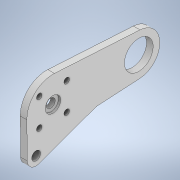
# Autodesk Inventor part: right_wall
Saved by Autodesk Inventor 2020 (Build 240168000, 168)
## iProperties
Created: 2024-02-19
Part Number: right_wall
Material: Типовые
Document SubType Name: Modeling
Designer: 4s
Density: 1 g/cm^3
Appearance: По умолчанию
Author: 4s
Autodesk Inventor part; units mm, degrees
ref_plane "YZ Plane" through (0, 0, 0) normal (1, 0, 0) x (0, 1, 0)
ref_plane "XZ Plane" through (0, 0, 0) normal (0, 1, 0) x (-1, 0, 0)
ref_plane "XY Plane" through (0, 0, 0) normal (0, 0, 1) x (1, 0, 0)
sketch "Эскиз1" plane through (0, 0, 0) normal (1, 0, 0) x (0, 1, 0)
  circle A0 centre (35.2311, -22.6062) radius 9.3
  circle A1 centre (0, -38.8201) radius 6.1
  circle A2 centre (0, 0) radius 4.85
  circle A3 centre (35.8147, -49.5529) radius 3.55
  line L0 (6.0968, -38.6237) -> (4.8475, 0.1562)
  line L1 (-4.8475, 0.1562) -> (-6.0968, -38.6237)
  line L2 (0, 0) -> (0, -38.8201) construction
  circle A4 centre (0, -38.8201) radius 6.5
  circle A5 centre (0, 0) radius 2
  circle A6 centre (0, -38.8201) radius 15 construction
  circle A7 centre (0, 0) radius 14 construction
  circle A8 centre (0, -38.8201) radius 9.5
  circle A9 centre (0, 0) radius 7
  line L3 (9.4833, -39.383) -> (11.7793, -0.6991)
  line L4 (-9.4833, -39.383) -> (-11.7793, -0.6991)
  circle A10 centre (0, 0) radius 8.8
  circle A11 centre (0, 0) radius 11.8
  point P0 (-7, 0)
  point P1 (-9.4833, -39.383)
  point P2 (-11.7793, -0.6991)
  dimension "d27" = 19
  dimension "d0" = 18.6
  dimension "d1" = 12.2
  dimension "d2" = 9.7
  dimension "d3" = 7.1
  dimension "d8" = 38.8201
  dimension "d13" = 38.8
  dimension "d14" = 38.8
  dimension "d23" = 13
  dimension "d24" = 4
  dimension "d25" = 30
  dimension "d26" = 28
  dimension "d28" = 14
  dimension "d31" = 17.6
  dimension "d32" = 3
  constraints: 10 centre point, 10 end point, 9 coincident, 4 point on circle, 4 tangent, 2 symmetric about line, 1 vertical, 8 other
  measures "d0" diameter of A0
  measures "d1" diameter of A1
  measures "d2" diameter of A2
  measures "d3" diameter of A3
  measures "d8" distance of L2.end L2.start
  measures "d13" distance of L0.start L0.end
  measures "d14" distance of L1.start L1.end
  measures "d23" diameter of A4
  measures "d24" diameter of A5
  measures "d25" diameter of A6
  measures "d26" diameter of A7
  measures "d28" diameter of A9
  measures "d31" diameter of A10
extrude "Выдавливание4" add sketch "Эскиз1" along normal blind 3 contours A4 L1 A8 L0 | L0 A8 L1 A4 | A8 L1 A11 L0 | L0 A11 L3 A8 | A8 L4 A11 L1 | A11 L1 A10 L0 | L0 A10 L1 A11 | A10 L1 A9 L0 | L0 A9 L1 A10 | A9 L1 A2 L0 | L0 A2 L1 A9 | A2
sketch "Эскиз4" plane through (0, 0, 0) normal (-1, 0, 0) x (0, 0, 1)
  circle A0 centre (-6.2, 6.2) radius 1.25
  circle A1 centre (0, 0) radius 2 construction
  circle A2 centre (-38.8201, 0) radius 6.5 construction
  arc A3 (-0.6991, -11.7793) -> (-0.6991, 11.7793) centre (0, 0) ccw construction
  line L0 (-39.383, 9.4833) -> (-0.6991, 11.7793) construction
  arc A4 (-39.383, 9.4833) -> (-39.383, -9.4833) centre (-38.8201, 0) ccw construction
  line L1 (-0.6991, -11.7793) -> (-39.383, -9.4833) construction
  line L2 (0, 0) -> (0, 11.8) construction
  arc A5 (-0.6991, -11.7793) -> (-0.6991, 11.7793) centre (0, 0) ccw construction
  line L3 (0, 0) -> (11.8, 0) construction
  circle A6 centre (6.2, 6.2) radius 1.25
  circle A7 centre (-6.2, -6.2) radius 1.25
  circle A8 centre (6.2, -6.2) radius 1.25
  dimension "d33" = 2.5
  dimension "d34" = 12.4
  dimension "d35" = 12.4
  constraints: 4 centre point, 4 end point, 3 point on circle, 3 symmetric about line, 1 vertical, 3 other
  measures "d33" diameter of A0
  measures "d34" distance of A6.centre A0.centre
  measures "d35" distance of A7.centre A0.centre
extrude "Выдавливание5" cut sketch "Эскиз4" against normal blind 3
sketch "Эскиз5" plane through (3, 0, 0) normal (1, 0, 0) x (0, 0, -1)
  circle A0 centre (0, 0) radius 3.5
  dimension "d38" = 7
  constraints: 1 centre point, 1 coincident
  measures "d38" diameter of A0
extrude "Выдавливание6" cut sketch "Эскиз5" against normal blind 1
sketch "Эскиз6" plane through (3, 0, 0) normal (1, 0, 0) x (0, 0, -1)
  circle A0 centre (0, -18) radius 2
  circle A1 centre (0, 0) radius 3.5 construction
  circle A2 centre (-6.2, -6.2) radius 1.25 construction
  circle A3 centre (-6.2, 6.2) radius 1.25 construction
  circle A4 centre (6.2, -6.2) radius 1.25 construction
  circle A5 centre (6.2, 6.2) radius 1.25 construction
  circle A6 centre (38.8201, 0) radius 6.5 construction
  line L0 (39.383, 9.4833) -> (0.6991, 11.7793) construction
  arc A7 (0.6991, 11.7793) -> (0.6991, -11.7793) centre (0, 0) ccw construction
  line L1 (0.6991, -11.7793) -> (39.383, -9.4833) construction
  arc A8 (39.383, -9.4833) -> (39.383, 9.4833) centre (38.8201, 0) ccw construction
  line L2 (0, 0) -> (0, -26.6004) construction
  circle A9 centre (0, 0) radius 14 construction
  line L3 (-10.6346, -5.1133) -> (-3.6049, -19.7333)
  arc A10 (0, -14) -> (-3.6049, -19.7333) centre (0, -18) ccw construction
  line L4 (2.8284, -20.8284) -> (12.5829, -11.0739)
  line L5 (0.6991, -11.7793) -> (39.383, -9.4833) construction
  arc A11 (2.8284, -20.8284) -> (0, -14) centre (0, -18) ccw construction
  arc A12 (-3.6049, -19.7333) -> (2.8284, -20.8284) centre (0, -18) ccw
  line L6 (-10.6346, -5.1133) -> (-9.9206, -5.1133)
  line L7 (-9.9206, -5.1133) -> (-6.5876, -8.9793)
  line L8 (-6.5876, -8.9793) -> (5.3497, -10.0676)
  line L9 (5.3497, -10.0676) -> (12.5829, -11.0739)
  dimension "d42" = 28
  dimension "d41" = 4
  dimension "d43" = 18
  dimension "d44" = 8
  dimension "d45" = 45
  constraints: 14 end point, 7 point on circle, 5 tangent, 4 centre point, 2 coincident, 2 point on line, 1 horizontal, 1 vertical, 1 vertical alignment, 2 other
  measures "d41" diameter of A0
  measures "d43" distance of point (0, 0) A0.centre
  measures "d44" diameter of A10
  measures "d45" angle of L2 L4
extrude "Выдавливание7" [suppressed]
sketch "Эскиз7" plane through (3, 0, 0) normal (1, 0, 0) x (0, 0, -1)
  line L0 (0, 0) -> (0, -29.4139) construction
  circle A0 centre (-7.6071, -16.3135) radius 2
  line L1 (-7.6071, -16.3135) -> (0, 0) construction
  circle A1 centre (0, 0) radius 14 construction
  circle A2 centre (0, 0) radius 18 construction
  arc A3 (-6.239, -20.0723) -> (-11.6068, -16.361) centre (-7.6071, -16.3135) ccw construction
  circle A4 centre (0, 0) radius 3.5 construction
  circle A5 centre (-6.2, -6.2) radius 1.25 construction
  circle A6 centre (-6.2, 6.2) radius 1.25 construction
  circle A7 centre (6.2, -6.2) radius 1.25 construction
  circle A8 centre (6.2, 6.2) radius 1.25 construction
  circle A9 centre (38.8201, 0) radius 6.5 construction
  line L2 (39.383, 9.4833) -> (0.6991, 11.7793) construction
  arc A10 (0.6991, 11.7793) -> (0.6991, -11.7793) centre (0, 0) ccw projected
  line L3 (0.6991, -11.7793) -> (39.383, -9.4833) projected
  arc A11 (39.383, -9.4833) -> (39.383, 9.4833) centre (38.8201, 0) ccw construction
  line L4 (-11.7992, -0.1399) -> (-11.6068, -16.361)
  line L5 (-6.239, -20.0723) -> (19.6335, -10.6555)
  line L6 (0.6991, -11.7793) -> (39.383, -9.4833) construction
  arc A12 (-11.6068, -16.361) -> (-6.239, -20.0723) centre (-7.6071, -16.3135) ccw
  point P0 (19.6335, -10.6555)
  dimension "d48" = 4
  dimension "d50" = 28
  dimension "d52" = 8
  dimension "d53" = 45
  dimension "d56" = 25
  dimension "d57" = 4
  constraints: 8 end point, 5 point on circle, 4 centre point, 3 coincident, 3 tangent, 1 point on line, 1 vertical, 3 other
  measures "d48" diameter of A0
  measures "d50" diameter of A1
  measures "d52" diameter of A3
  measures "d53" angle of L1 L5
  measures "d56" angle of L0 L1
extrude "Выдавливание8" add sketch "Эскиз7" against normal up to surface (3 mm away)
